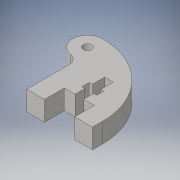
# Autodesk Inventor part: A8-0013
Saved by Autodesk Inventor 2016 SP2 (Build 200236200, 236)
## iProperties
Created: 2017-04-22
Part Number: A8-0013
Material: Generic
Document SubType Name: Modeling
Designer: EV
Density: 1 g/cm^3
Appearance: Default
Author: EV
Autodesk Inventor part; units mm, degrees
ref_plane "YZ Plane" through (0, 0, 0) normal (1, 0, 0) x (0, 1, 0)
sketch "Sketch1" plane through (0, 0, 0) normal (0, 1, 0) x (-1, 0, 0)
  line L0 (0, 0) -> (0, -4)
  line L1 (0, 0) -> (7.2, 0)
  line L2 (7.2, 0) -> (7.2, -8)
  line L3 (7.2, -8) -> (11.55, -8)
  line L4 (11.55, -8) -> (11.55, -12)
  line L5 (11.55, -12) -> (10.3, -12)
  line L6 (10.3, -12) -> (10.3, -15)
  line L7 (10.3, -15) -> (11.55, -15)
  line L8 (11.55, -15) -> (11.55, -20)
  line L9 (11.55, -20) -> (15.05, -20)
  line L10 (15.05, -20) -> (15.05, -15)
  line L11 (15.05, -15) -> (16.3, -15)
  line L12 (16.3, -15) -> (16.3, -12)
  line L13 (16.3, -12) -> (15.05, -12)
  line L14 (15.05, -8) -> (19.4, -8)
  line L15 (19.4, -8) -> (19.4, 0)
  line L16 (19.4, 0) -> (26.6, 0)
  line L17 (26.6, 0) -> (26.6, -17.1288)
  arc A0 (26.6, -17.1288) -> (29.96, -21.0773) centre (30.6, -17.1288) ccw
  line L18 (15.05, -12) -> (15.05, -8)
  arc A1 (0, -4) -> (29, -33) centre (29, -4) ccw
  arc A2 (29, -33) -> (29.96, -21.0773) centre (29, -27) ccw
  line L19 (29, -33) -> (0, -33) construction
  line L20 (0, -33) -> (0, -9.975) construction
  line L21 (13.3, -20) -> (13.3, 0) construction
  dimension "d0" = 7.2
  dimension "d1" = 12.2
  dimension "d2" = 4
  dimension "d3" = 3
  dimension "d4" = 5
  dimension "d5" = 3.5
  dimension "d6" = 6
  dimension "d7" = 8
  dimension "d8" = 7.2
  dimension "d9" = 33
  dimension "d10" = 35
  dimension "d11" = 6
  dimension "d12" = 4
  constraints: 44 end point, 13 perpendicular, 12 point on line, 6 point on circle, 5 tangent, 3 centre point, 3 collinear, 2 horizontal, 2 vertical, 1 midpoint
  measures "d0" distance of L0.start L1.end
  measures "d1" distance between parallel lines of L2 L15
  measures "d2" distance of L3.end L4.end
  measures "d3" distance of L5.end L6.end
  measures "d4" distance of L7.end L8.end
  measures "d5" distance between parallel lines of L18 L4
  measures "d6" distance between parallel lines of L6 L12
  measures "d7" distance of L1.end L2.end
  measures "d8" distance of L15.end L16.end
  measures "d9" distance from line of L1 L19.start
  measures "d11" radius of A2
  measures "d12" radius of A0
extrude "Extrusion1" add sketch "Sketch1" along normal blind 8
hole "Hole1" at (-29, 8, -27) direction (0, -1, 0) diameter 3.5 end through all
ref_plane "Work Plane1" through (0, 4, 0) normal (0, 1, 0) x (-1, 0, 0)
ref_plane "Work Plane2" through (-13.3, 0, -20) normal (-1, 0, 0) x (0, 0, 1)
equation "\"d24\" = 0.5 * THICKNESS"
equation "\"THICKNESS\" = 8"
body "Solid1"
